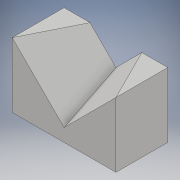
# Autodesk Inventor part: Part11
Saved by Autodesk Inventor 2017 (Build 210142000, 142)
## iProperties
Created: 2016-11-07
Part Number: Part11
Material: Generic
Document SubType Name: Modeling
Designer: s411888
Density: 1 g/cm^3
Appearance: Default
Author: s411888
Autodesk Inventor part; units mm, degrees
ref_plane "YZ Plane" through (0, 0, 0) normal (1, 0, 0) x (0, 1, 0)
ref_plane "XZ Plane" through (0, 0, 0) normal (0, 1, 0) x (-1, 0, 0)
ref_plane "XY Plane" through (0, 0, 0) normal (0, 0, 1) x (1, 0, 0)
sketch "Sketch1" plane through (0, 0, 0) normal (0, 0, 1) x (1, 0, 0)
  line L0 (-7.1627, 5.5131) -> (43.6373, 5.5131)
  line L1 (43.6373, 5.5131) -> (43.6373, -26.2369)
  line L2 (43.6373, -26.2369) -> (-7.1627, -26.2369)
  line L3 (-7.1627, -26.2369) -> (-7.1627, 5.5131)
  point P0 (0, 0)
  dimension "d0" = 50.8
  dimension "d1" = 31.75
  constraints: 8 end point, 2 parallel, 1 horizontal, 1 perpendicular
  measures "d0" distance of L1.end L2.end
  measures "d1" distance of L0.end L1.end
extrude "Extrusion1" add sketch "Sketch1" along normal blind 25.4
sketch "Sketch4" plane through (0, 0, 0) normal (0, 0, -1) x (-1, 0, 0)
  line L0 (-43.6373, 5.5131) -> (7.1627, 5.5131) projected
  line L1 (-43.6373, 5.5131) -> (-18.2373, -19.8869)
  line L2 (-18.2373, -19.8869) -> (7.1627, 5.5131)
  line L3 (7.1627, 5.5131) -> (-43.6373, 5.5131)
  line L4 (-43.6373, -26.2369) -> (7.1627, -26.2369) projected
  line L5 (7.1627, -26.2369) -> (7.1627, 5.5131) projected
  point P0 (0, 0)
  dimension "d10" = 6.35
  dimension "d11" = 25.4
  dimension "d12" = 0
  dimension "d13" = 0
  constraints: 6 end point, 2 point on line, 1 horizontal
  measures "d10" distance from line of L4 L1.end
  measures "d11" distance from line of L5 L1.end
  measures "d12" distance of L0.end L2.end
  measures "d13" distance of L0.start L1.start
sketch "Sketch6" plane through (0, 0, 25.4) normal (0, 0, 1) x (1, 0, 0)
  line L0 (43.6373, 5.5131) -> (-7.1627, 5.5131) projected
  line L1 (5.5373, 5.5131) -> (18.2373, -7.1869)
  line L2 (18.2373, -7.1869) -> (30.9373, 5.5131)
  line L3 (5.5373, 5.5131) -> (30.9373, 5.5131)
  line L4 (-7.1627, -26.2369) -> (43.6373, -26.2369) projected
  line L5 (43.6373, -26.2369) -> (43.6373, 5.5131) projected
  point P0 (0, 0)
  dimension "d14" = 12.7
  dimension "d15" = 12.7
  dimension "d16" = 19.05
  dimension "d17" = 25.4
  constraints: 6 end point, 2 point on line, 1 collinear
  measures "d14" distance of L0.end L1.start
  measures "d15" distance of L0.start L2.end
  measures "d16" distance from line of L4 L1.end
  measures "d17" distance from line of L5 L1.end
loft "Loft1" cut profiles "Sketch6", "Sketch4"
body "Solid1"
